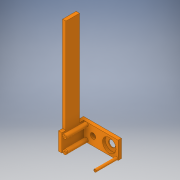
# Autodesk Inventor part: servo attachment claw
Saved by Autodesk Inventor 2017 (Build 210142000, 142)
## iProperties
Created: 2018-01-10
Part Number: servo attachment claw
Material: Generic
Document SubType Name: Modeling
Designer: Delta
Density: 1 g/cm^3
Appearance: Orange
Author: Delta
Autodesk Inventor part; units mm, degrees
ref_plane "YZ Plane" through (0, 0, 0) normal (1, 0, 0) x (0, 1, 0)
ref_plane "XZ Plane" through (0, 0, 0) normal (0, 1, 0) x (-1, 0, 0)
ref_plane "XY Plane" through (0, 0, 0) normal (0, 0, 1) x (1, 0, 0)
sketch "Sketch1" plane through (0, 0, 0) normal (0, 0, 1) x (1, 0, 0)
  line L0 (0, 0) -> (50.8, 0)
  line L1 (50.8, 0) -> (50.8, -33.02)
  line L2 (50.8, -33.02) -> (0, -33.02)
  line L3 (0, -33.02) -> (0, 0)
  dimension "d0" = 50.8
  dimension "d1" = 33.02
  constraints: 8 end point, 2 parallel, 1 horizontal, 1 perpendicular
  measures "d0" distance of L1.end L2.end
  measures "d1" distance of L0.end L1.end
extrude "Extrusion1" add sketch "Sketch1" along normal blind 6.35
sketch "Sketch2" plane through (0, 0, 6.35) normal (0, 0, 1) x (1, 0, 0)
  line L0 (50.8, 0) -> (0, 0) projected
  line L1 (0, 0) -> (0, -33.02) projected
  circle A0 centre (34.29, -16.51) radius 12.7
  point P0 (7.62, -16.51)
  dimension "d4" = 16.51
  dimension "d5" = 16.51
  dimension "d6" = 26.67
  dimension "d7" = 7.62
  dimension "d8" = 25.4
  constraints: 1 centre point, 1 coincident
  measures "d4" distance from line of point (7.62, -16.51) L0
  measures "d5" distance from line of L0 point (34.29, -16.51)
  measures "d6" distance of point (34.29, -16.51) point (7.62, -16.51)
  measures "d7" distance from line of L1 point (7.62, -16.51)
  measures "d8" diameter of A0
extrude "Extrusion2" cut sketch "Sketch2" against normal blind 5.08
sketch "Sketch3" plane through (34.29, -16.51, 1.27) normal (0, 0, 1) x (1, 0, 0)
  circle A0 centre (0, 0) radius 6.35
  point P0 (-34.29, 16.51)
  dimension "d11" = 12.7
  constraints: 1 centre point
  measures "d11" diameter of A0
extrude "Extrusion3" cut sketch "Sketch3" against normal blind 5.08
sketch "Sketch14" plane through (0, -33.02, 0) normal (-1, 0, 0) x (0, 0, 1)
  line L0 (0, 33.02) -> (6.35, 33.02)
  line L1 (6.35, 33.02) -> (6.35, 0)
  line L2 (6.35, 0) -> (0, 0)
  line L3 (0, 0) -> (0, 33.02)
  constraints: 8 end point, 2 parallel, 1 horizontal, 1 perpendicular
extrude "Extrusion14" add sketch "Sketch14" along normal blind 12.7
sketch "Sketch15" plane through (0, 0, 6.35) normal (0, 0, 1) x (1, 0, 0)
  line L0 (-12.7, -33.02) -> (-12.7, 0) projected
  line L1 (50.8, -33.02) -> (-12.7, -33.02) projected
  line L2 (50.8, 0) -> (-12.7, 0) projected
  circle A0 centre (-8.89, -3.81) radius 3.81
  circle A1 centre (-8.89, -29.21) radius 3.81
  circle A2 centre (-8.89, -29.21) radius 1.651
  circle A3 centre (-8.89, -3.81) radius 1.651
  point P0 (0, 0)
  dimension "d58" = 3.81
  dimension "d59" = 3.81
  dimension "d60" = 3.81
  dimension "d61" = 3.81
  dimension "d62" = 7.62
  dimension "d63" = 7.62
  dimension "d64" = 3.302
  dimension "d65" = 3.302
  constraints: 4 centre point, 4 coincident
  measures "d58" distance from line of L0 point (-8.89, -29.21)
  measures "d59" distance from line of point (-8.89, -29.21) L1
  measures "d60" distance from line of L2 point (-8.89, -3.81)
  measures "d61" distance from line of L0 point (-8.89, -3.81)
  measures "d62" diameter of A0
  measures "d63" diameter of A1
  measures "d64" diameter of A2
  measures "d65" diameter of A3
extrude "Extrusion15" add sketch "Sketch15" along normal blind 38.1 contours A1 | A0
sketch "Sketch16" plane through (0, 0, 6.35) normal (0, 0, 1) x (1, 0, 0)
  circle A0 centre (48.26, -30.48) radius 2.54
  line L0 (50.8, -33.02) -> (-8.89, -33.02) projected
  line L1 (50.8, -33.02) -> (50.8, 0) projected
  circle A1 centre (48.26, -30.48) radius 1.651
  point P0 (0, 0)
  dimension "d68" = 5.08
  dimension "d69" = 2.54
  dimension "d70" = 2.54
  dimension "d71" = 3.302
  constraints: 2 centre point, 1 coincident
  measures "d68" diameter of A0
  measures "d69" distance from line of L0 A0.centre
  measures "d70" distance from line of L1 A0.centre
  measures "d71" diameter of A1
extrude "Extrusion16" add sketch "Sketch16" along normal blind 38.1 contours A0
sketch "Sketch17" plane through (-8.89, -3.81, 44.45) normal (0, 0, 1) x (1, 0, 0)
  circle A0 centre (0, 0) radius 1.651 projected
  circle A1 centre (0, 0) radius 1.651
  circle A2 centre (0, 0) radius 3.81
  circle A3 centre (0, -25.396) radius 1.651
  circle A4 centre (0, -25.396) radius 3.81
  circle A5 centre (57.15, -26.67) radius 1.651 projected
  circle A6 centre (57.15, -26.67) radius 1.651
  circle A7 centre (57.15, -26.67) radius 2.54
  point P0 (8.89, 3.81)
  dimension "d74" = 3.302
  dimension "d75" = 7.62
  dimension "d76" = 3.302
  dimension "d77" = 7.62
  dimension "d78" = 5.08
  constraints: 6 centre point, 5 coincident
  measures "d74" diameter of A1
  measures "d75" diameter of A2
  measures "d76" diameter of A3
  measures "d77" diameter of A4
  measures "d78" diameter of A7
extrude "Extrusion17" add sketch "Sketch17" along normal blind 2.54
sketch "Sketch18" plane through (-12.7, -33.02, 0) normal (-1, 0, 0) x (0, 0, 1)
  line L0 (6.35, 3.81) -> (6.35, 0) projected
  line L1 (0, 33.02) -> (6.35, 33.02)
  line L2 (6.35, 33.02) -> (6.35, 0)
  line L3 (6.35, 0) -> (0, 0)
  line L4 (0, 0) -> (0, 33.02)
  constraints: 8 end point, 2 parallel, 1 horizontal, 1 perpendicular
extrude "Extrusion18" add sketch "Sketch18" along normal blind 12.7
sketch "Sketch20" plane through (-25.4, -33.02, 0) normal (-1, 0, 0) x (0, 0, 1)
  line L0 (0, 33.02) -> (0, 0) projected
  line L1 (0, 0) -> (6.35, 0) projected
  line L2 (0, 33.02) -> (6.35, 33.02)
  line L3 (6.35, 33.02) -> (6.35, 0)
  line L4 (6.35, 0) -> (0, 0)
  line L5 (0, 0) -> (0, 33.02)
  constraints: 8 end point, 2 parallel, 1 horizontal, 1 perpendicular
extrude "Extrusion20" cut sketch "Sketch20" against normal blind 5.08
sketch "Sketch21" plane through (0, 0, 6.35) normal (0, 0, 1) x (1, 0, 0)
  line L0 (-20.32, 0) -> (50.8, 0) projected
  line L1 (-20.32, 0) -> (-13.97, 0)
  line L2 (-13.97, 0) -> (-13.97, -33.02)
  line L3 (-13.97, -33.02) -> (-20.32, -33.02)
  line L4 (-20.32, -33.02) -> (-20.32, 0)
  point P0 (0, 0)
  dimension "d88" = 6.35
  dimension "d89" = 33.02
  constraints: 8 end point, 2 parallel, 1 horizontal, 1 perpendicular
  measures "d88" distance of L2.end L3.end
  measures "d89" distance of L1.end L2.end
extrude "Extrusion21" add sketch "Sketch21" along normal blind 40.64
sketch "Sketch23" plane through (50.8, 0, 6.35) normal (0, 1, 0) x (1, 0, 0)
  line L0 (-64.77, 0) -> (-64.77, -40.64) projected
  line L1 (-64.77, -7.62) -> (-71.12, -7.62)
  line L2 (-71.12, -7.62) -> (-71.12, -33.02)
  line L3 (-71.12, -33.02) -> (-64.77, -33.02)
  line L4 (-64.77, -33.02) -> (-64.77, -7.62)
  line L5 (-64.77, -40.64) -> (-71.12, -40.64) projected
  point P0 (-50.8, 6.35)
  dimension "d94" = 25.4
  dimension "d95" = 6.35
  dimension "d96" = 7.62
  constraints: 8 end point, 2 parallel, 1 horizontal, 1 perpendicular, 1 point on line
  measures "d94" distance of L2.end L1.end
  measures "d95" distance of L2.end L3.end
  measures "d96" distance between parallel lines of L5 L3
extrude "Extrusion23" add sketch "Sketch23" along normal blind 177.8
sketch "Sketch24" plane through (0, 0, 6.35) normal (0, 0, 1) x (1, 0, 0)
  circle A0 centre (3.81, -16.51) radius 5.08
  circle A1 centre (34.29, -16.51) radius 6.35 projected
  line L0 (48.26, -33.02) -> (-8.89, -33.02) projected
  point P0 (0, 0)
  dimension "d99" = 10.16
  dimension "d100" = 30.48
  dimension "d101" = 16.51
  constraints: 1 centre point
  measures "d99" diameter of A0
  measures "d100" distance of A1.centre A0.centre
  measures "d101" distance from line of L0 A0.centre
extrude "Extrusion24" cut sketch "Sketch24" against normal blind 25.4 contours A0
body "Solid1"
